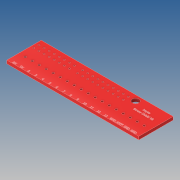
# Autodesk Inventor part: Arduino UNO R3 screw shield v2 board Left
Saved by Autodesk Inventor 2017 SP1 (Build 210196100, 196)
## iProperties
Created: 2022-11-07
Part Number: Arduino UNO R3 screw shield v2 board Left
Material: Generic
Document SubType Name: Modeling
Designer: Antonio
Density: 1 g/cm^3
Appearance: Rojo claro
Author: Antonio
Autodesk Inventor part; units mm, degrees
(part 1 of 2)
ref_plane "YZ Plane" through (0, 0, 0) normal (1, 0, 0) x (0, 1, 0)
ref_plane "XZ Plane" through (0, 0, 0) normal (0, 1, 0) x (-1, 0, 0)
ref_plane "XY Plane" through (0, 0, 0) normal (0, 0, 1) x (1, 0, 0)
sketch "Boceto1" plane through (0, 0, 0) normal (0, 0, 1) x (1, 0, 0)
  line L0 (0, 0) -> (66, 0)
  line L1 (66, 0) -> (66, 17.2)
  line L2 (66, 17.2) -> (0, 17.2)
  line L3 (0, 17.2) -> (0, 0)
  line L4 (0, 6) -> (66, 6) construction
  line L5 (3.3, 0) -> (3.3, 6) construction
  line L6 (6.8, 0) -> (6.8, 6) construction
  line L7 (10.3, 0) -> (10.3, 6) construction
  line L8 (13.8, 0) -> (13.8, 6) construction
  line L9 (17.3, 0) -> (17.3, 6) construction
  line L10 (20.8, 0) -> (20.8, 6) construction
  line L11 (24.3, 0) -> (24.3, 6) construction
  line L12 (27.8, 0) -> (27.8, 6) construction
  line L13 (31.3, 0) -> (31.3, 6) construction
  line L14 (34.8, 0) -> (34.8, 6) construction
  line L15 (38.3, 0) -> (38.3, 6) construction
  line L16 (41.8, 0) -> (41.8, 6) construction
  line L17 (45.3, 0) -> (45.3, 6) construction
  line L18 (48.8, 0) -> (48.8, 6) construction
  line L19 (52.3, 0) -> (52.3, 6) construction
  line L20 (55.8, 0) -> (55.8, 6) construction
  line L21 (59.3, 0) -> (59.3, 6) construction
  line L22 (62.8, 0) -> (62.8, 6) construction
  circle A0 centre (3.3, 6) radius 0.55
  circle A1 centre (6.8, 6) radius 0.55
  circle A2 centre (10.3, 6) radius 0.55
  circle A3 centre (13.8, 6) radius 0.55
  circle A4 centre (17.3, 6) radius 0.55
  circle A5 centre (20.8, 6) radius 0.55
  circle A6 centre (24.3, 6) radius 0.55
  circle A7 centre (27.8, 6) radius 0.55
  circle A8 centre (31.3, 6) radius 0.55
  circle A9 centre (34.8, 6) radius 0.55
  circle A10 centre (38.3, 6) radius 0.55
  circle A11 centre (41.8, 6) radius 0.55
  circle A12 centre (45.3, 6) radius 0.55
  circle A13 centre (48.8, 6) radius 0.55
  circle A14 centre (52.3, 6) radius 0.55
  circle A15 centre (55.8, 6) radius 0.55
  circle A16 centre (59.3, 6) radius 0.55
  circle A17 centre (62.8, 6) radius 0.55
  line L23 (0, 12) -> (66, 12) construction
  line L24 (0, 14.54) -> (66, 14.54) construction
  line L25 (1.54, 0) -> (1.54, 17.2) construction
  circle A18 centre (1.54, 14.54) radius 0.4
  circle A19 centre (4.08, 14.54) radius 0.4
  circle A20 centre (6.62, 14.54) radius 0.4
  circle A21 centre (9.16, 14.54) radius 0.4
  circle A22 centre (11.7, 14.54) radius 0.4
  circle A23 centre (14.24, 14.54) radius 0.4
  circle A24 centre (16.78, 14.54) radius 0.4
  circle A25 centre (19.32, 14.54) radius 0.4
  circle A26 centre (1.54, 12) radius 0.4
  circle A27 centre (4.08, 12) radius 0.4
  circle A28 centre (6.62, 12) radius 0.4
  circle A29 centre (9.16, 12) radius 0.4
  circle A30 centre (11.7, 12) radius 0.4
  circle A31 centre (14.24, 12) radius 0.4
  circle A32 centre (16.78, 12) radius 0.4
  circle A33 centre (19.32, 12) radius 0.4
  line L26 (19.32, 12) -> (19.32, 17.2) construction
  line L27 (23.384, 12) -> (23.384, 16.5) construction
  circle A34 centre (23.384, 14.54) radius 0.4
  circle A35 centre (25.924, 14.54) radius 0.4
  circle A36 centre (28.464, 14.54) radius 0.4
  circle A37 centre (31.004, 14.54) radius 0.4
  circle A38 centre (33.544, 14.54) radius 0.4
  circle A39 centre (36.084, 14.54) radius 0.4
  circle A40 centre (38.624, 14.54) radius 0.4
  circle A41 centre (41.164, 14.54) radius 0.4
  circle A42 centre (43.704, 14.54) radius 0.4
  circle A43 centre (46.244, 14.54) radius 0.4
  circle A44 centre (23.384, 12) radius 0.4
  circle A45 centre (25.924, 12) radius 0.4
  circle A46 centre (28.464, 12) radius 0.4
  circle A47 centre (31.004, 12) radius 0.4
  circle A48 centre (33.544, 12) radius 0.4
  circle A49 centre (36.084, 12) radius 0.4
  circle A50 centre (38.624, 12) radius 0.4
  circle A51 centre (41.164, 12) radius 0.4
  circle A52 centre (43.704, 12) radius 0.4
  circle A53 centre (46.244, 12) radius 0.4
  line L28 (46.244, 12) -> (46.244, 17.2) construction
  line L29 (50.76, 12) -> (50.76, 16.5) construction
  circle A54 centre (49.9, 14.54) radius 1.7
  line L30 (0, 0.2) -> (66, 0.2) construction
  line L31 (2.4235, 1.1897) -> (4.0751, 1.1897) construction
  line L32 (4.0751, 1.1897) -> (4.0751, 0.1897) construction
  line L33 (4.0751, 0.1897) -> (2.4235, 0.1897) construction
  line L34 (2.4235, 0.1897) -> (2.4235, 1.1897) construction
  line L35 (5.9424, 1.2002) -> (7.594, 1.2002) construction
  line L36 (7.594, 1.2002) -> (7.594, 0.2002) construction
  line L37 (7.594, 0.2002) -> (5.9424, 0.2002) construction
  line L38 (5.9424, 0.2002) -> (5.9424, 1.2002) construction
  line L39 (9.8961, 1.2406) -> (11.5477, 1.2406) construction
  line L40 (11.5477, 1.2406) -> (11.5477, 0.2406) construction
  line L41 (11.5477, 0.2406) -> (9.8961, 0.2406) construction
  line L42 (9.8961, 0.2406) -> (9.8961, 1.2406) construction
  line L43 (13.46, 0.221) -> (13.46, 1.221) construction
  line L44 (13.46, 1.221) -> (15.1116, 1.221) construction
  line L45 (15.1116, 1.221) -> (15.1116, 0.221) construction
  line L46 (15.1116, 0.221) -> (13.46, 0.221) construction
  line L47 (16.9339, 0.2315) -> (16.9339, 1.2315) construction
  line L48 (16.9339, 1.2315) -> (18.5855, 1.2315) construction
  line L49 (18.5855, 1.2315) -> (18.5855, 0.2315) construction
  line L50 (18.5855, 0.2315) -> (16.9339, 0.2315) construction
  line L51 (20.4229, 0.2269) -> (20.4229, 1.2269) construction
  line L52 (20.4229, 1.2269) -> (22.0744, 1.2269) construction
  line L53 (22.0744, 1.2269) -> (22.0744, 0.2269) construction
  line L54 (22.0744, 0.2269) -> (20.4229, 0.2269) construction
  line L55 (23.9268, 0.2373) -> (23.9268, 1.2373) construction
  line L56 (23.9268, 1.2373) -> (25.5783, 1.2373) construction
  line L57 (25.5783, 1.2373) -> (25.5783, 0.2373) construction
  line L58 (25.5783, 0.2373) -> (23.9268, 0.2373) construction
  line L59 (27.3857, 0.2627) -> (27.3857, 1.2627) construction
  line L60 (27.3857, 1.2627) -> (29.0372, 1.2627) construction
  line L61 (29.0372, 1.2627) -> (29.0372, 0.2627) construction
  line L62 (29.0372, 0.2627) -> (27.3857, 0.2627) construction
  line L63 (30.9196, 0.2732) -> (30.9196, 1.2732) construction
  line L64 (30.9196, 1.2732) -> (32.5711, 1.2732) construction
  line L65 (32.5711, 1.2732) -> (32.5711, 0.2732) construction
  line L66 (32.5711, 0.2732) -> (30.9196, 0.2732) construction
  line L67 (34.3935, 0.2386) -> (34.3935, 1.2386) construction
  line L68 (34.3935, 1.2386) -> (36.045, 1.2386) construction
  line L69 (36.045, 1.2386) -> (36.045, 0.2386) construction
  line L70 (36.045, 0.2386) -> (34.3935, 0.2386) construction
  line L71 (37.6275, 0.2041) -> (37.6275, 1.2041) construction
  line L72 (37.6275, 1.2041) -> (39.2791, 1.2041) construction
  line L73 (39.2791, 1.2041) -> (39.2791, 0.2041) construction
  line L74 (39.2791, 0.2041) -> (37.6275, 0.2041) construction
  line L75 (41.0265, 0.2295) -> (41.0265, 1.2295) construction
  line L76 (41.0265, 1.2295) -> (42.678, 1.2295) construction
  line L77 (42.678, 1.2295) -> (42.678, 0.2295) construction
  line L78 (42.678, 0.2295) -> (41.0265, 0.2295) construction
  line L79 (44.5754, 0.2249) -> (44.5754, 1.2249) construction
  line L80 (44.5754, 1.2249) -> (46.2269, 1.2249) construction
  line L81 (46.2269, 1.2249) -> (46.2269, 0.2249) construction
  line L82 (46.2269, 0.2249) -> (44.5754, 0.2249) construction
  line L83 (48.0793, 0.2204) -> (48.0793, 1.2204) construction
  line L84 (48.0793, 1.2204) -> (49.7308, 1.2204) construction
  line L85 (49.7308, 1.2204) -> (49.7308, 0.2204) construction
  line L86 (49.7308, 0.2204) -> (48.0793, 0.2204) construction
  line L87 (50.9534, 0.2458) -> (50.9534, 1.2458) construction
  line L88 (50.9534, 1.2458) -> (52.605, 1.2458) construction
  line L89 (52.605, 1.2458) -> (52.605, 0.2458) construction
  line L90 (52.605, 0.2458) -> (50.9534, 0.2458) construction
  line L91 (54.2025, 0.2263) -> (54.2025, 1.2263) construction
  line L92 (54.2025, 1.2263) -> (55.854, 1.2263) construction
  line L93 (55.854, 1.2263) -> (55.854, 0.2263) construction
  line L94 (55.854, 0.2263) -> (54.2025, 0.2263) construction
  line L95 (57.9208, 0.2413) -> (57.9208, 1.2413) construction
  line L96 (57.9208, 1.2413) -> (59.5724, 1.2413) construction
  line L97 (59.5724, 1.2413) -> (59.5724, 0.2413) construction
  line L98 (59.5724, 0.2413) -> (57.9208, 0.2413) construction
  line L99 (61.4098, 0.2067) -> (61.4098, 1.2067) construction
  line L100 (61.4098, 1.2067) -> (64.5007, 1.2067) construction
  line L101 (64.5007, 1.2067) -> (64.5007, 0.2067) construction
  line L102 (64.5007, 0.2067) -> (61.4098, 0.2067) construction
  line L103 (55.5956, 13.2313) -> (59.0259, 13.2313) construction
  line L104 (59.0259, 13.2313) -> (59.0259, 11.9104) construction
  line L105 (59.0259, 11.9104) -> (55.5956, 11.9104) construction
  line L106 (55.5956, 11.9104) -> (55.5956, 13.2313) construction
  line L107 (52.8192, 11.2798) -> (62.9552, 11.2798) construction
  line L108 (62.9552, 11.2798) -> (62.9552, 10.186) construction
  line L109 (62.9552, 10.186) -> (52.8192, 10.186) construction
  line L110 (52.8192, 10.186) -> (52.8192, 11.2798) construction
  line L111 (56.3087, 12.1867) -> (56.1426, 12.1867)
  line L112 (56.1426, 12.1867) -> (55.8638, 12.549)
  line L113 (55.8638, 12.549) -> (55.8136, 12.5004)
  line L114 (55.8136, 12.5004) -> (55.8136, 12.1867)
  line L115 (55.8136, 12.1867) -> (55.6872, 12.1867)
  line L116 (55.6872, 12.1867) -> (55.6872, 13.2313)
  line L117 (55.6872, 13.2313) -> (55.8136, 13.2313)
  line L118 (55.8136, 13.2313) -> (55.8136, 12.6203)
  line L119 (55.8136, 12.6203) -> (56.1102, 12.9371)
  line L120 (56.1102, 12.9371) -> (56.2674, 12.9371)
  line L121 (56.2674, 12.9371) -> (55.9595, 12.6235)
  line L122 (55.9595, 12.6235) -> (56.3087, 12.1867)
  spline S0 degree 2 poles (56.6977, 12.1697) (56.5178, 12.1697) (56.3201, 12.3715) (56.3201, 12.5579) knots 0 0 0 1 2 2 2
  spline S1 degree 2 poles (56.3201, 12.5579) (56.3201, 12.741) (56.5121, 12.9582) (56.6669, 12.9582) knots 0 0 0 1 2 2 2
  spline S2 degree 2 poles (56.6669, 12.9582) (56.7366, 12.9582) (56.8444, 12.9177) (56.8841, 12.8747) knots 0 0 0 1 2 2 2
  spline S3 degree 2 poles (56.8841, 12.8747) (56.9246, 12.8318) (56.9676, 12.7078) (56.9676, 12.6179) knots 0 0 0 1 2 2 2
  line L123 (56.9676, 12.6179) -> (56.9676, 12.549)
  line L124 (56.9676, 12.549) -> (56.4481, 12.549)
  spline S4 degree 2 poles (56.4481, 12.549) (56.4481, 12.4185) (56.5794, 12.2799) (56.6961, 12.2799) knots 0 0 0 1 2 2 2
  spline S5 degree 2 poles (56.6961, 12.2799) (56.7374, 12.2799) (56.8176, 12.2986) (56.8501, 12.3132) knots 0 0 0 1 2 2 2
  spline S6 degree 2 poles (56.8501, 12.3132) (56.8841, 12.3294) (56.9311, 12.3577) (56.9465, 12.3707) knots 0 0 0 1 2 2 2
  line L125 (56.9465, 12.3707) -> (56.9538, 12.3707)
  line L126 (56.9538, 12.3707) -> (56.9538, 12.2329)
  spline S7 degree 2 poles (56.9538, 12.2329) (56.9319, 12.224) (56.8655, 12.1981) (56.8395, 12.1908) knots 0 0 0 1 2 2 2
  spline S8 degree 2 poles (56.8395, 12.1908) (56.8031, 12.1803) (56.7431, 12.1697) (56.6977, 12.1697) knots 0 0 0 1 2 2 2
  spline S9 degree 2 poles (56.8444, 12.6454) (56.8428, 12.6965) (56.8217, 12.771) (56.8014, 12.7961) knots 0 0 0 1 2 2 2
  spline S10 degree 2 poles (56.8014, 12.7961) (56.7796, 12.8245) (56.7107, 12.8545) (56.6596, 12.8545) knots 0 0 0 1 2 2 2
  spline S11 degree 2 poles (56.6596, 12.8545) (56.6094, 12.8545) (56.5389, 12.8245) (56.5097, 12.7953) knots 0 0 0 1 2 2 2
  spline S12 degree 2 poles (56.5097, 12.7953) (56.4813, 12.7653) (56.4522, 12.6932) (56.4481, 12.6454) knots 0 0 0 1 2 2 2
  line L127 (56.4481, 12.6454) -> (56.8444, 12.6454)
  line L128 (57.6847, 12.9371) -> (57.2812, 11.9104)
  line L129 (57.2812, 11.9104) -> (57.1458, 11.9104)
  line L130 (57.1458, 11.9104) -> (57.2804, 12.2232)
  line L131 (57.2804, 12.2232) -> (57.0081, 12.9371)
  line L132 (57.0081, 12.9371) -> (57.1442, 12.9371)
  line L133 (57.1442, 12.9371) -> (57.3492, 12.3812)
  line L134 (57.3492, 12.3812) -> (57.5535, 12.9371)
  line L135 (57.5535, 12.9371) -> (57.6847, 12.9371)
  spline S13 degree 2 poles (58.1061, 12.1697) (57.9262, 12.1697) (57.7285, 12.3715) (57.7285, 12.5579) knots 0 0 0 1 2 2 2
  spline S14 degree 2 poles (57.7285, 12.5579) (57.7285, 12.741) (57.9206, 12.9582) (58.0753, 12.9582) knots 0 0 0 1 2 2 2
  spline S15 degree 2 poles (58.0753, 12.9582) (58.145, 12.9582) (58.2528, 12.9177) (58.2925, 12.8747) knots 0 0 0 1 2 2 2
  spline S16 degree 2 poles (58.2925, 12.8747) (58.333, 12.8318) (58.376, 12.7078) (58.376, 12.6179) knots 0 0 0 1 2 2 2
  line L136 (58.376, 12.6179) -> (58.376, 12.549)
  line L137 (58.376, 12.549) -> (57.8565, 12.549)
  spline S17 degree 2 poles (57.8565, 12.549) (57.8565, 12.4185) (57.9878, 12.2799) (58.1045, 12.2799) knots 0 0 0 1 2 2 2
  spline S18 degree 2 poles (58.1045, 12.2799) (58.1458, 12.2799) (58.2261, 12.2986) (58.2585, 12.3132) knots 0 0 0 1 2 2 2
  spline S19 degree 2 poles (58.2585, 12.3132) (58.2925, 12.3294) (58.3395, 12.3577) (58.3549, 12.3707) knots 0 0 0 1 2 2 2
  line L138 (58.3549, 12.3707) -> (58.3622, 12.3707)
  line L139 (58.3622, 12.3707) -> (58.3622, 12.2329)
  spline S20 degree 2 poles (58.3622, 12.2329) (58.3403, 12.224) (58.2739, 12.1981) (58.248, 12.1908) knots 0 0 0 1 2 2 2
  spline S21 degree 2 poles (58.248, 12.1908) (58.2115, 12.1803) (58.1515, 12.1697) (58.1061, 12.1697) knots 0 0 0 1 2 2 2
  spline S22 degree 2 poles (58.2528, 12.6454) (58.2512, 12.6965) (58.2301, 12.771) (58.2099, 12.7961) knots 0 0 0 1 2 2 2
  spline S23 degree 2 poles (58.2099, 12.7961) (58.188, 12.8245) (58.1191, 12.8545) (58.0681, 12.8545) knots 0 0 0 1 2 2 2
  spline S24 degree 2 poles (58.0681, 12.8545) (58.0178, 12.8545) (57.9473, 12.8245) (57.9181, 12.7953) knots 0 0 0 1 2 2 2
  spline S25 degree 2 poles (57.9181, 12.7953) (57.8898, 12.7653) (57.8606, 12.6932) (57.8565, 12.6454) knots 0 0 0 1 2 2 2
  line L140 (57.8565, 12.6454) -> (58.2528, 12.6454)
  spline S26 degree 2 poles (58.7066, 12.1689) (58.6313, 12.1689) (58.5008, 12.2094) (58.4578, 12.2321) knots 0 0 0 1 2 2 2
  line L141 (58.4578, 12.2321) -> (58.4578, 12.3739)
  line L142 (58.4578, 12.3739) -> (58.4643, 12.3739)
  spline S27 degree 2 poles (58.4643, 12.3739) (58.4805, 12.361) (58.5243, 12.3302) (58.5608, 12.3132) knots 0 0 0 1 2 2 2
  spline S28 degree 2 poles (58.5608, 12.3132) (58.5924, 12.2978) (58.6702, 12.2751) (58.7115, 12.2751) knots 0 0 0 1 2 2 2
  spline S29 degree 2 poles (58.7115, 12.2751) (58.7415, 12.2751) (58.8104, 12.2888) (58.8266, 12.3002) knots 0 0 0 1 2 2 2
  spline S30 degree 2 poles (58.8266, 12.3002) (58.8501, 12.3156) (58.8711, 12.3504) (58.8711, 12.3861) knots 0 0 0 1 2 2 2
  spline S31 degree 2 poles (58.8711, 12.3861) (58.8711, 12.4307) (58.8225, 12.4769) (58.7601, 12.4923) knots 0 0 0 1 2 2 2
  spline S32 degree 2 poles (58.7601, 12.4923) (58.7358, 12.4979) (58.658, 12.5141) (58.6248, 12.523) knots 0 0 0 1 2 2 2
  spline S33 degree 2 poles (58.6248, 12.523) (58.5389, 12.5482) (58.4611, 12.6519) (58.4611, 12.7256) knots 0 0 0 1 2 2 2
  spline S34 degree 2 poles (58.4611, 12.7256) (58.4611, 12.8277) (58.6142, 12.955) (58.7407, 12.955) knots 0 0 0 1 2 2 2
  spline S35 degree 2 poles (58.7407, 12.955) (58.8031, 12.955) (58.9295, 12.9242) (58.9724, 12.9007) knots 0 0 0 1 2 2 2
  line L143 (58.9724, 12.9007) -> (58.9724, 12.7653)
  line L144 (58.9724, 12.7653) -> (58.9659, 12.7653)
  spline S36 degree 2 poles (58.9659, 12.7653) (58.9173, 12.8042) (58.799, 12.8488) (58.7382, 12.8488) knots 0 0 0 1 2 2 2
  spline S37 degree 2 poles (58.7382, 12.8488) (58.6758, 12.8488) (58.5899, 12.7961) (58.5899, 12.7435) knots 0 0 0 1 2 2 2
  spline S38 degree 2 poles (58.5899, 12.7435) (58.5899, 12.6957) (58.641, 12.6495) (58.6977, 12.6349) knots 0 0 0 1 2 2 2
  spline S39 degree 2 poles (58.6977, 12.6349) (58.7253, 12.6276) (58.795, 12.613) (58.833, 12.6041) knots 0 0 0 1 2 2 2
  spline S40 degree 2 poles (58.833, 12.6041) (58.9157, 12.583) (59, 12.4866) (59, 12.4031) knots 0 0 0 1 2 2 2
  spline S41 degree 2 poles (59, 12.4031) (59, 12.3545) (58.9619, 12.2686) (58.9246, 12.237) knots 0 0 0 1 2 2 2
  spline S42 degree 2 poles (58.9246, 12.237) (58.8849, 12.2038) (58.7836, 12.1689) (58.7066, 12.1689) knots 0 0 0 1 2 2 2
  spline S43 degree 2 poles (53.1993, 10.2174) (53.0907, 10.2174) (52.9383, 10.2627) (52.8711, 10.2952) knots 0 0 0 1 2 2 2
  line L145 (52.8711, 10.2952) -> (52.8711, 10.4621)
  line L146 (52.8711, 10.4621) -> (52.8808, 10.4621)
  spline S44 degree 2 poles (52.8808, 10.4621) (52.9464, 10.4005) (53.1126, 10.3324) (53.1895, 10.3324) knots 0 0 0 1 2 2 2
  spline S45 degree 2 poles (53.1895, 10.3324) (53.2998, 10.3324) (53.4124, 10.424) (53.4124, 10.4994) knots 0 0 0 1 2 2 2
  spline S46 degree 2 poles (53.4124, 10.4994) (53.4124, 10.5593) (53.3532, 10.6339) (53.2892, 10.6525) knots 0 0 0 1 2 2 2
  spline S47 degree 2 poles (53.2892, 10.6525) (53.243, 10.6655) (53.166, 10.6833) (53.1085, 10.6979) knots 0 0 0 1 2 2 2
  spline S48 degree 2 poles (53.1085, 10.6979) (53.0566, 10.7117) (52.9748, 10.753) (52.9432, 10.7862) knots 0 0 0 1 2 2 2
  spline S49 degree 2 poles (52.9432, 10.7862) (52.9124, 10.8195) (52.8784, 10.9086) (52.8784, 10.967) knots 0 0 0 1 2 2 2
  spline S50 degree 2 poles (52.8784, 10.967) (52.8784, 11.0885) (53.068, 11.253) (53.2147, 11.253) knots 0 0 0 1 2 2 2
  spline S51 degree 2 poles (53.2147, 11.253) (53.2989, 11.253) (53.4481, 11.2198) (53.5121, 11.1882) knots 0 0 0 1 2 2 2
  line L147 (53.5121, 11.1882) -> (53.5121, 11.0294)
  line L148 (53.5121, 11.0294) -> (53.5024, 11.0294)
  spline S52 degree 2 poles (53.5024, 11.0294) (53.4545, 11.0731) (53.3054, 11.1379) (53.2236, 11.1379) knots 0 0 0 1 2 2 2
  spline S53 degree 2 poles (53.2236, 11.1379) (53.1312, 11.1379) (53.0169, 11.0512) (53.0169, 10.9807) knots 0 0 0 1 2 2 2
  spline S54 degree 2 poles (53.0169, 10.9807) (53.0169, 10.9175) (53.0842, 10.8422) (53.1474, 10.8251) knots 0 0 0 1 2 2 2
  spline S55 degree 2 poles (53.1474, 10.8251) (53.1895, 10.8138) (53.3119, 10.7846) (53.3524, 10.7725) knots 0 0 0 1 2 2 2
  spline S56 degree 2 poles (53.3524, 10.7725) (53.4554, 10.7409) (53.551, 10.6136) (53.551, 10.5204) knots 0 0 0 1 2 2 2
  spline S57 degree 2 poles (53.551, 10.5204) (53.551, 10.4613) (53.5032, 10.3478) (53.4602, 10.3081) knots 0 0 0 1 2 2 2
  spline S58 degree 2 poles (53.4602, 10.3081) (53.4124, 10.2644) (53.2908, 10.2174) (53.1993, 10.2174) knots 0 0 0 1 2 2 2
  spline S59 degree 2 poles (53.9748, 10.2182) (53.897, 10.2182) (53.7682, 10.266) (53.722, 10.3146) knots 0 0 0 1 2 2 2
  spline S60 degree 2 poles (53.722, 10.3146) (53.6758, 10.3624) (53.6247, 10.5099) (53.6247, 10.6088) knots 0 0 0 1 2 2 2
  spline S61 degree 2 poles (53.6247, 10.6088) (53.6247, 10.7076) (53.6774, 10.8519) (53.722, 10.9005) knots 0 0 0 1 2 2 2
  spline S62 degree 2 poles (53.722, 10.9005) (53.7665, 10.9499) (53.8986, 11.0026) (53.9748, 11.0026) knots 0 0 0 1 2 2 2
  spline S63 degree 2 poles (53.9748, 11.0026) (54.0364, 11.0026) (54.1515, 10.9678) (54.196, 10.9451) knots 0 0 0 1 2 2 2
  line L149 (54.196, 10.9451) -> (54.196, 10.8033)
  line L150 (54.196, 10.8033) -> (54.1887, 10.8033)
  spline S64 degree 2 poles (54.1887, 10.8033) (54.175, 10.8146) (54.1328, 10.8438) (54.1028, 10.8592) knots 0 0 0 1 2 2 2
  spline S65 degree 2 poles (54.1028, 10.8592) (54.0761, 10.8721) (54.0048, 10.8924) (53.9724, 10.8924) knots 0 0 0 1 2 2 2
  spline S66 degree 2 poles (53.9724, 10.8924) (53.8743, 10.8924) (53.7552, 10.7441) (53.7552, 10.6088) knots 0 0 0 1 2 2 2
  spline S67 degree 2 poles (53.7552, 10.6088) (53.7552, 10.4767) (53.8703, 10.3284) (53.9724, 10.3284) knots 0 0 0 1 2 2 2
  spline S68 degree 2 poles (53.9724, 10.3284) (54.034, 10.3284) (54.1458, 10.3794) (54.1887, 10.4191) knots 0 0 0 1 2 2 2
  line L151 (54.1887, 10.4191) -> (54.196, 10.4191)
  line L152 (54.196, 10.4191) -> (54.196, 10.2773)
  spline S69 degree 2 poles (54.196, 10.2773) (54.1774, 10.2684) (54.1207, 10.2433) (54.098, 10.2376) knots 0 0 0 1 2 2 2
  spline S70 degree 2 poles (54.098, 10.2376) (54.0656, 10.2279) (54.0145, 10.2182) (53.9748, 10.2182) knots 0 0 0 1 2 2 2
  line L153 (54.709, 10.8503) -> (54.7025, 10.8503)
  spline S71 degree 2 poles (54.7025, 10.8503) (54.6879, 10.8543) (54.6563, 10.8559) (54.6344, 10.8559) knots 0 0 0 1 2 2 2
  spline S72 degree 2 poles (54.6344, 10.8559) (54.5834, 10.8559) (54.4829, 10.8114) (54.4375, 10.7676) knots 0 0 0 1 2 2 2
  line L154 (54.4375, 10.7676) -> (54.4375, 10.2352)
  line L155 (54.4375, 10.2352) -> (54.3111, 10.2352)
  line L156 (54.3111, 10.2352) -> (54.3111, 10.9856)
  line L157 (54.3111, 10.9856) -> (54.4375, 10.9856)
  line L158 (54.4375, 10.9856) -> (54.4375, 10.8738)
  spline S73 degree 2 poles (54.4375, 10.8738) (54.5064, 10.9353) (54.6093, 10.9856) (54.6579, 10.9856) knots 0 0 0 1 2 2 2
  spline S74 degree 2 poles (54.6579, 10.9856) (54.6774, 10.9856) (54.6968, 10.984) (54.709, 10.9815) knots 0 0 0 1 2 2 2
  line L159 (54.709, 10.9815) -> (54.709, 10.8503)
  spline S75 degree 2 poles (55.1328, 10.2182) (54.9529, 10.2182) (54.7552, 10.42) (54.7552, 10.6063) knots 0 0 0 1 2 2 2
  spline S76 degree 2 poles (54.7552, 10.6063) (54.7552, 10.7895) (54.9472, 11.0067) (55.102, 11.0067) knots 0 0 0 1 2 2 2
  spline S77 degree 2 poles (55.102, 11.0067) (55.1717, 11.0067) (55.2795, 10.9661) (55.3192, 10.9232) knots 0 0 0 1 2 2 2
  spline S78 degree 2 poles (55.3192, 10.9232) (55.3597, 10.8802) (55.4027, 10.7563) (55.4027, 10.6663) knots 0 0 0 1 2 2 2
  line L160 (55.4027, 10.6663) -> (55.4027, 10.5974)
  line L161 (55.4027, 10.5974) -> (54.8832, 10.5974)
  spline S79 degree 2 poles (54.8832, 10.5974) (54.8832, 10.467) (55.0145, 10.3284) (55.1312, 10.3284) knots 0 0 0 1 2 2 2
  spline S80 degree 2 poles (55.1312, 10.3284) (55.1725, 10.3284) (55.2528, 10.347) (55.2852, 10.3616) knots 0 0 0 1 2 2 2
  spline S81 degree 2 poles (55.2852, 10.3616) (55.3192, 10.3778) (55.3662, 10.4062) (55.3816, 10.4191) knots 0 0 0 1 2 2 2
  line L162 (55.3816, 10.4191) -> (55.3889, 10.4191)
  line L163 (55.3889, 10.4191) -> (55.3889, 10.2814)
  spline S82 degree 2 poles (55.3889, 10.2814) (55.367, 10.2725) (55.3006, 10.2465) (55.2746, 10.2392) knots 0 0 0 1 2 2 2
  spline S83 degree 2 poles (55.2746, 10.2392) (55.2382, 10.2287) (55.1782, 10.2182) (55.1328, 10.2182) knots 0 0 0 1 2 2 2
  spline S84 degree 2 poles (55.2795, 10.6939) (55.2779, 10.7449) (55.2568, 10.8195) (55.2366, 10.8446) knots 0 0 0 1 2 2 2
  spline S85 degree 2 poles (55.2366, 10.8446) (55.2147, 10.8729) (55.1458, 10.9029) (55.0947, 10.9029) knots 0 0 0 1 2 2 2
  spline S86 degree 2 poles (55.0947, 10.9029) (55.0445, 10.9029) (54.974, 10.8729) (54.9448, 10.8438) knots 0 0 0 1 2 2 2
  spline S87 degree 2 poles (54.9448, 10.8438) (54.9165, 10.8138) (54.8873, 10.7417) (54.8832, 10.6939) knots 0 0 0 1 2 2 2
  line L164 (54.8832, 10.6939) -> (55.2795, 10.6939)
  line L165 (56.44, 10.9856) -> (56.2495, 10.2352)
  line L166 (56.2495, 10.2352) -> (56.1328, 10.2352)
  line L167 (56.1328, 10.2352) -> (55.9497, 10.8138)
  line L168 (55.9497, 10.8138) -> (55.7673, 10.2352)
  line L169 (55.7673, 10.2352) -> (55.6515, 10.2352)
  line L170 (55.6515, 10.2352) -> (55.4594, 10.9856)
  line L171 (55.4594, 10.9856) -> (55.5907, 10.9856)
  line L172 (55.5907, 10.9856) -> (55.7236, 10.4046)
  line L173 (55.7236, 10.4046) -> (55.9011, 10.9856)
  line L174 (55.9011, 10.9856) -> (56.0056, 10.9856)
  line L175 (56.0056, 10.9856) -> (56.1879, 10.4046)
  line L176 (56.1879, 10.4046) -> (56.3127, 10.9856)
  line L177 (56.3127, 10.9856) -> (56.44, 10.9856)
  spline S88 degree 2 poles (57.269, 10.2174) (57.1604, 10.2174) (57.008, 10.2627) (56.9408, 10.2952) knots 0 0 0 1 2 2 2
  line L178 (56.9408, 10.2952) -> (56.9408, 10.4621)
  line L179 (56.9408, 10.4621) -> (56.9505, 10.4621)
  spline S89 degree 2 poles (56.9505, 10.4621) (57.0161, 10.4005) (57.1823, 10.3324) (57.2592, 10.3324) knots 0 0 0 1 2 2 2
  spline S90 degree 2 poles (57.2592, 10.3324) (57.3695, 10.3324) (57.4821, 10.424) (57.4821, 10.4994) knots 0 0 0 1 2 2 2
  spline S91 degree 2 poles (57.4821, 10.4994) (57.4821, 10.5593) (57.4229, 10.6339) (57.3589, 10.6525) knots 0 0 0 1 2 2 2
  spline S92 degree 2 poles (57.3589, 10.6525) (57.3127, 10.6655) (57.2357, 10.6833) (57.1782, 10.6979) knots 0 0 0 1 2 2 2
  spline S93 degree 2 poles (57.1782, 10.6979) (57.1263, 10.7117) (57.0445, 10.753) (57.0129, 10.7862) knots 0 0 0 1 2 2 2
  spline S94 degree 2 poles (57.0129, 10.7862) (56.9821, 10.8195) (56.9481, 10.9086) (56.9481, 10.967) knots 0 0 0 1 2 2 2
  spline S95 degree 2 poles (56.9481, 10.967) (56.9481, 11.0885) (57.1377, 11.253) (57.2844, 11.253) knots 0 0 0 1 2 2 2
  spline S96 degree 2 poles (57.2844, 11.253) (57.3686, 11.253) (57.5177, 11.2198) (57.5818, 11.1882) knots 0 0 0 1 2 2 2
  line L180 (57.5818, 11.1882) -> (57.5818, 11.0294)
  line L181 (57.5818, 11.0294) -> (57.572, 11.0294)
  spline S97 degree 2 poles (57.572, 11.0294) (57.5242, 11.0731) (57.3751, 11.1379) (57.2933, 11.1379) knots 0 0 0 1 2 2 2
  spline S98 degree 2 poles (57.2933, 11.1379) (57.2009, 11.1379) (57.0866, 11.0512) (57.0866, 10.9807) knots 0 0 0 1 2 2 2
  spline S99 degree 2 poles (57.0866, 10.9807) (57.0866, 10.9175) (57.1539, 10.8422) (57.2171, 10.8251) knots 0 0 0 1 2 2 2
  spline S100 degree 2 poles (57.2171, 10.8251) (57.2592, 10.8138) (57.3816, 10.7846) (57.4221, 10.7725) knots 0 0 0 1 2 2 2
  spline S101 degree 2 poles (57.4221, 10.7725) (57.525, 10.7409) (57.6207, 10.6136) (57.6207, 10.5204) knots 0 0 0 1 2 2 2
  spline S102 degree 2 poles (57.6207, 10.5204) (57.6207, 10.4613) (57.5729, 10.3478) (57.5299, 10.3081) knots 0 0 0 1 2 2 2
  spline S103 degree 2 poles (57.5299, 10.3081) (57.4821, 10.2644) (57.3605, 10.2174) (57.269, 10.2174) knots 0 0 0 1 2 2 2
  line L182 (58.3354, 10.2352) -> (58.209, 10.2352)
  line L183 (58.209, 10.2352) -> (58.209, 10.6631)
  spline S104 degree 2 poles (58.209, 10.6631) (58.209, 10.7149) (58.1993, 10.8041) (58.1847, 10.8308) knots 0 0 0 1 2 2 2
  spline S105 degree 2 poles (58.1847, 10.8308) (58.1693, 10.8592) (58.1142, 10.8867) (58.0672, 10.8867) knots 0 0 0 1 2 2 2
  spline S106 degree 2 poles (58.0672, 10.8867) (58.0202, 10.8867) (57.9205, 10.8365) (57.8727, 10.796) knots 0 0 0 1 2 2 2
  line L184 (57.8727, 10.796) -> (57.8727, 10.2352)
  line L185 (57.8727, 10.2352) -> (57.7463, 10.2352)
  line L186 (57.7463, 10.2352) -> (57.7463, 11.2798)
  line L187 (57.7463, 11.2798) -> (57.8727, 11.2798)
  line L188 (57.8727, 11.2798) -> (57.8727, 10.9021)
  spline S107 degree 2 poles (57.8727, 10.9021) (57.9294, 10.9532) (58.0388, 11.0067) (58.1004, 11.0067) knots 0 0 0 1 2 2 2
  spline S108 degree 2 poles (58.1004, 11.0067) (58.2106, 11.0067) (58.3354, 10.8608) (58.3354, 10.7222) knots 0 0 0 1 2 2 2
  line L189 (58.3354, 10.7222) -> (58.3354, 10.2352)
  line L190 (58.6417, 10.2352) -> (58.5153, 10.2352)
  line L191 (58.5153, 10.2352) -> (58.5153, 10.9856)
  line L192 (58.5153, 10.9856) -> (58.6417, 10.9856)
  line L193 (58.6417, 10.9856) -> (58.6417, 10.2352)
  line L194 (58.6507, 11.1104) -> (58.5072, 11.1104)
  line L195 (58.5072, 11.1104) -> (58.5072, 11.2417)
  line L196 (58.5072, 11.2417) -> (58.6507, 11.2417)
  line L197 (58.6507, 11.2417) -> (58.6507, 11.1104)
  spline S109 degree 2 poles (59.1531, 10.2182) (58.9732, 10.2182) (58.7754, 10.42) (58.7754, 10.6063) knots 0 0 0 1 2 2 2
  spline S110 degree 2 poles (58.7754, 10.6063) (58.7754, 10.7895) (58.9675, 11.0067) (59.1223, 11.0067) knots 0 0 0 1 2 2 2
  spline S111 degree 2 poles (59.1223, 11.0067) (59.192, 11.0067) (59.2998, 10.9661) (59.3395, 10.9232) knots 0 0 0 1 2 2 2
  spline S112 degree 2 poles (59.3395, 10.9232) (59.38, 10.8802) (59.4229, 10.7563) (59.4229, 10.6663) knots 0 0 0 1 2 2 2
  line L198 (59.4229, 10.6663) -> (59.4229, 10.5974)
  line L199 (59.4229, 10.5974) -> (58.9035, 10.5974)
  spline S113 degree 2 poles (58.9035, 10.5974) (58.9035, 10.467) (59.0348, 10.3284) (59.1515, 10.3284) knots 0 0 0 1 2 2 2
  spline S114 degree 2 poles (59.1515, 10.3284) (59.1928, 10.3284) (59.273, 10.347) (59.3054, 10.3616) knots 0 0 0 1 2 2 2
  spline S115 degree 2 poles (59.3054, 10.3616) (59.3395, 10.3778) (59.3865, 10.4062) (59.4019, 10.4191) knots 0 0 0 1 2 2 2
  line L200 (59.4019, 10.4191) -> (59.4092, 10.4191)
  line L201 (59.4092, 10.4191) -> (59.4092, 10.2814)
  spline S116 degree 2 poles (59.4092, 10.2814) (59.3873, 10.2725) (59.3208, 10.2465) (59.2949, 10.2392) knots 0 0 0 1 2 2 2
  spline S117 degree 2 poles (59.2949, 10.2392) (59.2584, 10.2287) (59.1985, 10.2182) (59.1531, 10.2182) knots 0 0 0 1 2 2 2
  spline S118 degree 2 poles (59.2998, 10.6939) (59.2981, 10.7449) (59.2771, 10.8195) (59.2568, 10.8446) knots 0 0 0 1 2 2 2
  spline S119 degree 2 poles (59.2568, 10.8446) (59.2349, 10.8729) (59.166, 10.9029) (59.115, 10.9029) knots 0 0 0 1 2 2 2
  spline S120 degree 2 poles (59.115, 10.9029) (59.0648, 10.9029) (58.9942, 10.8729) (58.9651, 10.8438) knots 0 0 0 1 2 2 2
  spline S121 degree 2 poles (58.9651, 10.8438) (58.9367, 10.8138) (58.9075, 10.7417) (58.9035, 10.6939) knots 0 0 0 1 2 2 2
  line L202 (58.9035, 10.6939) -> (59.2998, 10.6939)
  line L203 (59.6798, 10.2352) -> (59.5534, 10.2352)
  line L204 (59.5534, 10.2352) -> (59.5534, 11.2798)
  line L205 (59.5534, 11.2798) -> (59.6798, 11.2798)
  line L206 (59.6798, 11.2798) -> (59.6798, 10.2352)
  line L207 (60.4424, 10.2352) -> (60.316, 10.2352)
  line L208 (60.316, 10.2352) -> (60.316, 10.3114)
  spline S122 degree 2 poles (60.316, 10.3114) (60.2868, 10.2871) (60.2438, 10.2546) (60.2147, 10.2409) knots 0 0 0 1 2 2 2
  spline S123 degree 2 poles (60.2147, 10.2409) (60.1879, 10.2279) (60.1304, 10.2141) (60.0923, 10.2141) knots 0 0 0 1 2 2 2
  spline S124 degree 2 poles (60.0923, 10.2141) (60.0307, 10.2141) (59.927, 10.2652) (59.8905, 10.3146) knots 0 0 0 1 2 2 2
  spline S125 degree 2 poles (59.8905, 10.3146) (59.8541, 10.364) (59.8135, 10.5099) (59.8135, 10.6047) knots 0 0 0 1 2 2 2
  spline S126 degree 2 poles (59.8135, 10.6047) (59.8135, 10.7036) (59.8646, 10.8478) (59.9092, 10.9021) knots 0 0 0 1 2 2 2
  spline S127 degree 2 poles (59.9092, 10.9021) (59.9505, 10.9507) (60.0664, 11.0067) (60.1304, 11.0067) knots 0 0 0 1 2 2 2
  spline S128 degree 2 poles (60.1304, 11.0067) (60.1863, 11.0067) (60.2698, 10.9815) (60.316, 10.9556) knots 0 0 0 1 2 2 2
  line L209 (60.316, 10.9556) -> (60.316, 11.2798)
  line L210 (60.316, 11.2798) -> (60.4424, 11.2798)
  line L211 (60.4424, 11.2798) -> (60.4424, 10.2352)
  line L212 (60.316, 10.4175) -> (60.316, 10.8511)
  spline S129 degree 2 poles (60.316, 10.8511) (60.269, 10.8738) (60.1944, 10.8908) (60.1515, 10.8908) knots 0 0 0 1 2 2 2
  spline S130 degree 2 poles (60.1515, 10.8908) (60.0542, 10.8908) (59.944, 10.7449) (59.944, 10.6071) knots 0 0 0 1 2 2 2
  spline S131 degree 2 poles (59.944, 10.6071) (59.944, 10.4742) (60.0283, 10.3341) (60.1215, 10.3341) knots 0 0 0 1 2 2 2
  spline S132 degree 2 poles (60.1215, 10.3341) (60.1709, 10.3341) (60.2714, 10.3794) (60.316, 10.4175) knots 0 0 0 1 2 2 2
  line L213 (61.79, 11.2352) -> (61.4456, 10.2352)
  line L214 (61.4456, 10.2352) -> (61.3022, 10.2352)
  line L215 (61.3022, 10.2352) -> (60.9578, 11.2352)
  line L216 (60.9578, 11.2352) -> (61.1004, 11.2352)
  line L217 (61.1004, 11.2352) -> (61.3776, 10.4046)
  line L218 (61.3776, 10.4046) -> (61.6547, 11.2352)
  line L219 (61.6547, 11.2352) -> (61.79, 11.2352)
  line L220 (62.474, 10.2352) -> (61.8573, 10.2352)
  line L221 (61.8573, 10.2352) -> (61.8573, 10.377)
  spline S133 degree 2 poles (61.8573, 10.377) (61.9237, 10.4394) (62.0421, 10.5553) (62.0988, 10.6177) knots 0 0 0 1 2 2 2
  spline S134 degree 2 poles (62.0988, 10.6177) (62.213, 10.7433) (62.2965, 10.894) (62.2965, 10.9742) knots 0 0 0 1 2 2 2
  spline S135 degree 2 poles (62.2965, 10.9742) (62.2965, 11.0164) (62.2706, 11.0796) (62.2471, 11.0999) knots 0 0 0 1 2 2 2
  spline S136 degree 2 poles (62.2471, 11.0999) (62.2236, 11.1201) (62.162, 11.1404) (62.1247, 11.1404) knots 0 0 0 1 2 2 2
  spline S137 degree 2 poles (62.1247, 11.1404) (62.0891, 11.1404) (62.0161, 11.1225) (61.9829, 11.1088) knots 0 0 0 1 2 2 2
  spline S138 degree 2 poles (61.9829, 11.1088) (61.9545, 11.0974) (61.9019, 11.065) (61.8857, 11.0537) knots 0 0 0 1 2 2 2
  line L222 (61.8857, 11.0537) -> (61.8784, 11.0537)
  line L223 (61.8784, 11.0537) -> (61.8784, 11.1963)
  spline S139 degree 2 poles (61.8784, 11.1963) (61.9197, 11.2165) (62.068, 11.2563) (62.1344, 11.2563) knots 0 0 0 1 2 2 2
  spline S140 degree 2 poles (62.1344, 11.2563) (62.2746, 11.2563) (62.4327, 11.108) (62.4327, 10.9815) knots 0 0 0 1 2 2 2
  spline S141 degree 2 poles (62.4327, 10.9815) (62.4327, 10.9224) (62.4051, 10.8235) (62.3808, 10.7814) knots 0 0 0 1 2 2 2
  spline S142 degree 2 poles (62.3808, 10.7814) (62.3565, 10.7376) (62.286, 10.6517) (62.2471, 10.6104) knots 0 0 0 1 2 2 2
  spline S143 degree 2 poles (62.2471, 10.6104) (62.1839, 10.5415) (62.0291, 10.394) (61.9829, 10.3511) knots 0 0 0 1 2 2 2
  line L224 (61.9829, 10.3511) -> (62.474, 10.3511)
  line L225 (62.474, 10.3511) -> (62.474, 10.2352)
  spline S144 degree 2 poles (61.93, 0.1694) (61.8239, 0.1694) (61.648, 0.2343) (61.5848, 0.2999) knots 0 0 0 1 2 2 2
  spline S145 degree 2 poles (61.5848, 0.2999) (61.5216, 0.3663) (61.4543, 0.5625) (61.4543, 0.6897) knots 0 0 0 1 2 2 2
  spline S146 degree 2 poles (61.4543, 0.6897) (61.4543, 0.8104) (61.5224, 1.0017) (61.5856, 1.0698) knots 0 0 0 1 2 2 2
  spline S147 degree 2 poles (61.5856, 1.0698) (61.6464, 1.1354) (61.8247, 1.2067) (61.9308, 1.2067) knots 0 0 0 1 2 2 2
  spline S148 degree 2 poles (61.9308, 1.2067) (61.9819, 1.2067) (62.0743, 1.1921) (62.1164, 1.1792) knots 0 0 0 1 2 2 2
  spline S149 degree 2 poles (62.1164, 1.1792) (62.1504, 1.1694) (62.2331, 1.1338) (62.2582, 1.1208) knots 0 0 0 1 2 2 2
  line L226 (62.2582, 1.1208) -> (62.2582, 0.9604)
  line L227 (62.2582, 0.9604) -> (62.2469, 0.9604)
  spline S150 degree 2 poles (62.2469, 0.9604) (62.2217, 0.9822) (62.1691, 1.0219) (62.1204, 1.0446) knots 0 0 0 1 2 2 2
  spline S151 degree 2 poles (62.1204, 1.0446) (62.0799, 1.0649) (61.9754, 1.0916) (61.9154, 1.0916) knots 0 0 0 1 2 2 2
  spline S152 degree 2 poles (61.9154, 1.0916) (61.7712, 1.0916) (61.5929, 0.8745) (61.5929, 0.6937) knots 0 0 0 1 2 2 2
  spline S153 degree 2 poles (61.5929, 0.6937) (61.5929, 0.5933) (61.6399, 0.4425) (61.6845, 0.3907) knots 0 0 0 1 2 2 2
  spline S154 degree 2 poles (61.6845, 0.3907) (61.7274, 0.3388) (61.849, 0.2845) (61.9251, 0.2845) knots 0 0 0 1 2 2 2
  spline S155 degree 2 poles (61.9251, 0.2845) (61.9811, 0.2845) (62.0929, 0.3007) (62.131, 0.3169) knots 0 0 0 1 2 2 2
  line L228 (62.131, 0.3169) -> (62.131, 0.5754)
  line L229 (62.131, 0.5754) -> (61.8992, 0.5754)
  line L230 (61.8992, 0.5754) -> (61.8992, 0.6921)
  line L231 (61.8992, 0.6921) -> (62.2623, 0.6921)
  line L232 (62.2623, 0.6921) -> (62.2623, 0.2553)
  spline S156 degree 2 poles (62.2623, 0.2553) (62.2371, 0.244) (62.1512, 0.2091) (62.1148, 0.1986) knots 0 0 0 1 2 2 2
  spline S157 degree 2 poles (62.1148, 0.1986) (62.0653, 0.184) (61.9859, 0.1694) (61.93, 0.1694) knots 0 0 0 1 2 2 2
  line L233 (63.1448, 0.1889) -> (62.9957, 0.1889)
  line L234 (62.9957, 0.1889) -> (62.5532, 1.0511)
  line L235 (62.5532, 1.0511) -> (62.5532, 0.1889)
  line L236 (62.5532, 0.1889) -> (62.4292, 0.1889)
  line L237 (62.4292, 0.1889) -> (62.4292, 1.1889)
  line L238 (62.4292, 1.1889) -> (62.618, 1.1889)
  line L239 (62.618, 1.1889) -> (63.0208, 0.3971)
  line L240 (63.0208, 0.3971) -> (63.0208, 1.1889)
  line L241 (63.0208, 1.1889) -> (63.1448, 1.1889)
  line L242 (63.1448, 1.1889) -> (63.1448, 0.1889)
  spline S158 degree 2 poles (64.1358, 0.6881) (64.1358, 0.5511) (64.0248, 0.3307) (63.9316, 0.2691) knots 0 0 0 1 2 2 2
  spline S159 degree 2 poles (63.9316, 0.2691) (63.8555, 0.2213) (63.6991, 0.1889) (63.5775, 0.1889) knots 0 0 0 1 2 2 2
  line L243 (63.5775, 0.1889) -> (63.3474, 0.1889)
  line L244 (63.3474, 0.1889) -> (63.3474, 1.1889)
  line L245 (63.3474, 1.1889) -> (63.5751, 1.1889)
  spline S160 degree 2 poles (63.5751, 1.1889) (63.7161, 1.1889) (63.8765, 1.1467) (63.9333, 1.1095) knots 0 0 0 1 2 2 2
  spline S161 degree 2 poles (63.9333, 1.1095) (64.0297, 1.0454) (64.1358, 0.8339) (64.1358, 0.6881) knots 0 0 0 1 2 2 2
  spline S162 degree 2 poles (63.9973, 0.6897) (63.9973, 0.8048) (63.9211, 0.9676) (63.8457, 1.0138) knots 0 0 0 1 2 2 2
  spline S163 degree 2 poles (63.8457, 1.0138) (63.7922, 1.0454) (63.6715, 1.0738) (63.5816, 1.0738) knots 0 0 0 1 2 2 2
  line L246 (63.5816, 1.0738) -> (63.4803, 1.0738)
  line L247 (63.4803, 1.0738) -> (63.4803, 0.304)
  line L248 (63.4803, 0.304) -> (63.5816, 0.304)
  spline S164 degree 2 poles (63.5816, 0.304) (63.6699, 0.304) (63.8036, 0.3323) (63.8579, 0.3704) knots 0 0 0 1 2 2 2
  spline S165 degree 2 poles (63.8579, 0.3704) (63.9276, 0.4174) (63.9973, 0.573) (63.9973, 0.6897) knots 0 0 0 1 2 2 2
  spline S166 degree 2 poles (58.4411, 0.204) (58.3349, 0.204) (58.1591, 0.2688) (58.0959, 0.3344) knots 0 0 0 1 2 2 2
  spline S167 degree 2 poles (58.0959, 0.3344) (58.0327, 0.4009) (57.9654, 0.597) (57.9654, 0.7242) knots 0 0 0 1 2 2 2
  spline S168 degree 2 poles (57.9654, 0.7242) (57.9654, 0.845) (58.0335, 1.0362) (58.0967, 1.1043) knots 0 0 0 1 2 2 2
  spline S169 degree 2 poles (58.0967, 1.1043) (58.1575, 1.1699) (58.3358, 1.2413) (58.4419, 1.2413) knots 0 0 0 1 2 2 2
  spline S170 degree 2 poles (58.4419, 1.2413) (58.493, 1.2413) (58.5853, 1.2267) (58.6275, 1.2137) knots 0 0 0 1 2 2 2
  spline S171 degree 2 poles (58.6275, 1.2137) (58.6615, 1.204) (58.7442, 1.1683) (58.7693, 1.1554) knots 0 0 0 1 2 2 2
  line L249 (58.7693, 1.1554) -> (58.7693, 0.9949)
  line L250 (58.7693, 0.9949) -> (58.758, 0.9949)
  spline S172 degree 2 poles (58.758, 0.9949) (58.7328, 1.0168) (58.6802, 1.0565) (58.6315, 1.0792) knots 0 0 0 1 2 2 2
  spline S173 degree 2 poles (58.6315, 1.0792) (58.591, 1.0994) (58.4865, 1.1262) (58.4265, 1.1262) knots 0 0 0 1 2 2 2
  spline S174 degree 2 poles (58.4265, 1.1262) (58.2823, 1.1262) (58.104, 0.909) (58.104, 0.7283) knots 0 0 0 1 2 2 2
  spline S175 degree 2 poles (58.104, 0.7283) (58.104, 0.6278) (58.151, 0.4771) (58.1956, 0.4252) knots 0 0 0 1 2 2 2
  spline S176 degree 2 poles (58.1956, 0.4252) (58.2385, 0.3733) (58.3601, 0.319) (58.4362, 0.319) knots 0 0 0 1 2 2 2
  spline S177 degree 2 poles (58.4362, 0.319) (58.4922, 0.319) (58.604, 0.3353) (58.6421, 0.3515) knots 0 0 0 1 2 2 2
  line L251 (58.6421, 0.3515) -> (58.6421, 0.61)
  line L252 (58.6421, 0.61) -> (58.4103, 0.61)
  line L253 (58.4103, 0.61) -> (58.4103, 0.7267)
  line L254 (58.4103, 0.7267) -> (58.7734, 0.7267)
  line L255 (58.7734, 0.7267) -> (58.7734, 0.2899)
  spline S178 degree 2 poles (58.7734, 0.2899) (58.7482, 0.2785) (58.6623, 0.2437) (58.6259, 0.2332) knots 0 0 0 1 2 2 2
  spline S179 degree 2 poles (58.6259, 0.2332) (58.5764, 0.2186) (58.497, 0.204) (58.4411, 0.204) knots 0 0 0 1 2 2 2
  line L256 (59.6558, 0.2234) -> (59.5067, 0.2234)
  line L257 (59.5067, 0.2234) -> (59.0643, 1.0857)
  line L258 (59.0643, 1.0857) -> (59.0643, 0.2234)
  line L259 (59.0643, 0.2234) -> (58.9403, 0.2234)
  line L260 (58.9403, 0.2234) -> (58.9403, 1.2234)
  line L261 (58.9403, 1.2234) -> (59.1291, 1.2234)
  line L262 (59.1291, 1.2234) -> (59.5319, 0.4317)
  line L263 (59.5319, 0.4317) -> (59.5319, 1.2234)
  line L264 (59.5319, 1.2234) -> (59.6558, 1.2234)
  line L265 (59.6558, 1.2234) -> (59.6558, 0.2234)
  spline S180 degree 2 poles (60.6469, 0.7226) (60.6469, 0.5857) (60.5359, 0.3652) (60.4427, 0.3037) knots 0 0 0 1 2 2 2
  spline S181 degree 2 poles (60.4427, 0.3037) (60.3665, 0.2558) (60.2101, 0.2234) (60.0886, 0.2234) knots 0 0 0 1 2 2 2
  line L266 (60.0886, 0.2234) -> (59.8584, 0.2234)
  line L267 (59.8584, 0.2234) -> (59.8584, 1.2234)
  line L268 (59.8584, 1.2234) -> (60.0862, 1.2234)
  spline S182 degree 2 poles (60.0862, 1.2234) (60.2272, 1.2234) (60.3876, 1.1813) (60.4443, 1.144) knots 0 0 0 1 2 2 2
  spline S183 degree 2 poles (60.4443, 1.144) (60.5408, 1.08) (60.6469, 0.8685) (60.6469, 0.7226) knots 0 0 0 1 2 2 2
  spline S184 degree 2 poles (60.5084, 0.7242) (60.5084, 0.8393) (60.4322, 1.0022) (60.3568, 1.0484) knots 0 0 0 1 2 2 2
  spline S185 degree 2 poles (60.3568, 1.0484) (60.3033, 1.08) (60.1826, 1.1084) (60.0926, 1.1084) knots 0 0 0 1 2 2 2
  line L269 (60.0926, 1.1084) -> (59.9913, 1.1084)
  line L270 (59.9913, 1.1084) -> (59.9913, 0.3385)
  line L271 (59.9913, 0.3385) -> (60.0926, 0.3385)
  spline S186 degree 2 poles (60.0926, 0.3385) (60.181, 0.3385) (60.3147, 0.3669) (60.369, 0.4049) knots 0 0 0 1 2 2 2
  spline S187 degree 2 poles (60.369, 0.4049) (60.4387, 0.452) (60.5084, 0.6075) (60.5084, 0.7242) knots 0 0 0 1 2 2 2
  line L272 (54.196, 0.2263) -> (54.5331, 1.2263)
  line L273 (54.5331, 1.2263) -> (54.6968, 1.2263)
  line L274 (54.6968, 1.2263) -> (55.0339, 0.2263)
  line L275 (55.0339, 0.2263) -> (54.8937, 0.2263)
  line L276 (54.8937, 0.2263) -> (54.803, 0.5058)
  line L277 (54.803, 0.5058) -> (54.4213, 0.5058)
  line L278 (54.4213, 0.5058) -> (54.3305, 0.2263)
  line L279 (54.3305, 0.2263) -> (54.196, 0.2263)
  line L280 (54.7665, 0.6193) -> (54.6117, 1.0901)
  line L281 (54.6117, 1.0901) -> (54.4577, 0.6193)
  line L282 (54.4577, 0.6193) -> (54.7665, 0.6193)
  line L283 (55.9026, 0.2263) -> (55.73, 0.2263)
  line L284 (55.73, 0.2263) -> (55.414, 0.6242)
  line L285 (55.414, 0.6242) -> (55.2616, 0.6242)
  line L286 (55.2616, 0.6242) -> (55.2616, 0.2263)
  line L287 (55.2616, 0.2263) -> (55.1287, 0.2263)
  line L288 (55.1287, 0.2263) -> (55.1287, 1.2263)
  line L289 (55.1287, 1.2263) -> (55.3864, 1.2263)
  spline S188 degree 2 poles (55.3864, 1.2263) (55.4723, 1.2263) (55.5882, 1.2076) (55.6409, 1.1736) knots 0 0 0 1 2 2 2
  spline S189 degree 2 poles (55.6409, 1.1736) (55.6936, 1.1396) (55.7543, 1.0334) (55.7543, 0.9548) knots 0 0 0 1 2 2 2
  spline S190 degree 2 poles (55.7543, 0.9548) (55.7543, 0.8454) (55.6425, 0.6971) (55.5469, 0.6614) knots 0 0 0 1 2 2 2
  line L290 (55.5469, 0.6614) -> (55.9026, 0.2263)
  spline S191 degree 2 poles (55.6158, 0.9443) (55.6158, 0.988) (55.585, 1.0553) (55.5525, 1.0772) knots 0 0 0 1 2 2 2
  spline S192 degree 2 poles (55.5525, 1.0772) (55.5242, 1.0958) (55.4488, 1.1112) (55.3937, 1.1112) knots 0 0 0 1 2 2 2
  line L291 (55.3937, 1.1112) -> (55.2616, 1.1112)
  line L292 (55.2616, 1.1112) -> (55.2616, 0.7352)
  line L293 (55.2616, 0.7352) -> (55.3783, 0.7352)
  spline S193 degree 2 poles (55.3783, 0.7352) (55.4359, 0.7352) (55.5274, 0.7554) (55.559, 0.787) knots 0 0 0 1 2 2 2
  spline S194 degree 2 poles (55.559, 0.787) (55.5882, 0.8146) (55.6158, 0.8924) (55.6158, 0.9443) knots 0 0 0 1 2 2 2
  line L294 (56.5801, 1.1079) -> (56.1149, 1.1079)
  line L295 (56.1149, 1.1079) -> (56.1149, 0.8259)
  line L296 (56.1149, 0.8259) -> (56.5606, 0.8259)
  line L297 (56.5606, 0.8259) -> (56.5606, 0.7076)
  line L298 (56.5606, 0.7076) -> (56.1149, 0.7076)
  line L299 (56.1149, 0.7076) -> (56.1149, 0.2263)
  line L300 (56.1149, 0.2263) -> (55.982, 0.2263)
  line L301 (55.982, 0.2263) -> (55.982, 1.2263)
  line L302 (55.982, 1.2263) -> (56.5801, 1.2263)
  line L303 (56.5801, 1.2263) -> (56.5801, 1.1079)
  line L304 (57.2973, 1.1079) -> (56.8321, 1.1079)
  line L305 (56.8321, 1.1079) -> (56.8321, 0.8259)
  line L306 (56.8321, 0.8259) -> (57.2778, 0.8259)
  line L307 (57.2778, 0.8259) -> (57.2778, 0.7076)
  line L308 (57.2778, 0.7076) -> (56.8321, 0.7076)
  line L309 (56.8321, 0.7076) -> (56.8321, 0.2263)
  line L310 (56.8321, 0.2263) -> (56.6992, 0.2263)
  line L311 (56.6992, 0.2263) -> (56.6992, 1.2263)
  line L312 (56.6992, 1.2263) -> (57.2973, 1.2263)
  line L313 (57.2973, 1.2263) -> (57.2973, 1.1079)
  spline S195 degree 2 poles (51.4737, 0.2085) (51.3675, 0.2085) (51.1917, 0.2734) (51.1285, 0.339) knots 0 0 0 1 2 2 2
  spline S196 degree 2 poles (51.1285, 0.339) (51.0653, 0.4055) (50.998, 0.6016) (50.998, 0.7288) knots 0 0 0 1 2 2 2
  spline S197 degree 2 poles (50.998, 0.7288) (50.998, 0.8495) (51.0661, 1.0408) (51.1293, 1.1089) knots 0 0 0 1 2 2 2
  spline S198 degree 2 poles (51.1293, 1.1089) (51.1901, 1.1745) (51.3684, 1.2458) (51.4745, 1.2458) knots 0 0 0 1 2 2 2
  spline S199 degree 2 poles (51.4745, 1.2458) (51.5256, 1.2458) (51.618, 1.2312) (51.6601, 1.2183) knots 0 0 0 1 2 2 2
  spline S200 degree 2 poles (51.6601, 1.2183) (51.6941, 1.2085) (51.7768, 1.1729) (51.8019, 1.1599) knots 0 0 0 1 2 2 2
  line L314 (51.8019, 1.1599) -> (51.8019, 0.9995)
  line L315 (51.8019, 0.9995) -> (51.7906, 0.9995)
  spline S201 degree 2 poles (51.7906, 0.9995) (51.7654, 1.0213) (51.7128, 1.061) (51.6641, 1.0837) knots 0 0 0 1 2 2 2
  spline S202 degree 2 poles (51.6641, 1.0837) (51.6236, 1.104) (51.5191, 1.1307) (51.4591, 1.1307) knots 0 0 0 1 2 2 2
  spline S203 degree 2 poles (51.4591, 1.1307) (51.3149, 1.1307) (51.1366, 0.9136) (51.1366, 0.7328) knots 0 0 0 1 2 2 2
  spline S204 degree 2 poles (51.1366, 0.7328) (51.1366, 0.6324) (51.1836, 0.4816) (51.2282, 0.4298) knots 0 0 0 1 2 2 2
  spline S205 degree 2 poles (51.2282, 0.4298) (51.2711, 0.3779) (51.3927, 0.3236) (51.4688, 0.3236) knots 0 0 0 1 2 2 2
  spline S206 degree 2 poles (51.4688, 0.3236) (51.5248, 0.3236) (51.6366, 0.3398) (51.6747, 0.356) knots 0 0 0 1 2 2 2
  line L316 (51.6747, 0.356) -> (51.6747, 0.6145)
  line L317 (51.6747, 0.6145) -> (51.4429, 0.6145)
  line L318 (51.4429, 0.6145) -> (51.4429, 0.7312)
  line L319 (51.4429, 0.7312) -> (51.806, 0.7312)
  line L320 (51.806, 0.7312) -> (51.806, 0.2944)
  spline S207 degree 2 poles (51.806, 0.2944) (51.7808, 0.2831) (51.6949, 0.2482) (51.6585, 0.2377) knots 0 0 0 1 2 2 2
  spline S208 degree 2 poles (51.6585, 0.2377) (51.609, 0.2231) (51.5296, 0.2085) (51.4737, 0.2085) knots 0 0 0 1 2 2 2
  line L321 (52.6885, 0.228) -> (52.5393, 0.228)
  line L322 (52.5393, 0.228) -> (52.0969, 1.0902)
  line L323 (52.0969, 1.0902) -> (52.0969, 0.228)
  line L324 (52.0969, 0.228) -> (51.9729, 0.228)
  line L325 (51.9729, 0.228) -> (51.9729, 1.228)
  line L326 (51.9729, 1.228) -> (52.1617, 1.228)
  line L327 (52.1617, 1.228) -> (52.5645, 0.4363)
  line L328 (52.5645, 0.4363) -> (52.5645, 1.228)
  line L329 (52.5645, 1.228) -> (52.6885, 1.228)
  line L330 (52.6885, 1.228) -> (52.6885, 0.228)
  spline S209 degree 2 poles (53.6795, 0.7272) (53.6795, 0.5902) (53.5685, 0.3698) (53.4753, 0.3082) knots 0 0 0 1 2 2 2
  spline S210 degree 2 poles (53.4753, 0.3082) (53.3992, 0.2604) (53.2428, 0.228) (53.1212, 0.228) knots 0 0 0 1 2 2 2
  line L331 (53.1212, 0.228) -> (52.891, 0.228)
  line L332 (52.891, 0.228) -> (52.891, 1.228)
  line L333 (52.891, 1.228) -> (53.1188, 1.228)
  spline S211 degree 2 poles (53.1188, 1.228) (53.2598, 1.228) (53.4202, 1.1858) (53.4769, 1.1486) knots 0 0 0 1 2 2 2
  spline S212 degree 2 poles (53.4769, 1.1486) (53.5734, 1.0846) (53.6795, 0.873) (53.6795, 0.7272) knots 0 0 0 1 2 2 2
  spline S213 degree 2 poles (53.541, 0.7288) (53.541, 0.8439) (53.4648, 1.0068) (53.3894, 1.0529) knots 0 0 0 1 2 2 2
  spline S214 degree 2 poles (53.3894, 1.0529) (53.3359, 1.0846) (53.2152, 1.1129) (53.1252, 1.1129) knots 0 0 0 1 2 2 2
  line L334 (53.1252, 1.1129) -> (53.0239, 1.1129)
  line L335 (53.0239, 1.1129) -> (53.0239, 0.3431)
  line L336 (53.0239, 0.3431) -> (53.1252, 0.3431)
  spline S215 degree 2 poles (53.1252, 0.3431) (53.2136, 0.3431) (53.3473, 0.3714) (53.4016, 0.4095) knots 0 0 0 1 2 2 2
  spline S216 degree 2 poles (53.4016, 0.4095) (53.4713, 0.4565) (53.541, 0.6121) (53.541, 0.7288) knots 0 0 0 1 2 2 2
  line L337 (48.7187, 0.1993) -> (48.2308, 0.1993)
  line L338 (48.2308, 0.1993) -> (48.2308, 0.3014)
  line L339 (48.2308, 0.3014) -> (48.4123, 0.3014)
  line L340 (48.4123, 0.3014) -> (48.4123, 0.9716)
  line L341 (48.4123, 0.9716) -> (48.2308, 0.9716)
  line L342 (48.2308, 0.9716) -> (48.2308, 1.0632)
  spline S217 degree 2 poles (48.2308, 1.0632) (48.3337, 1.0632) (48.431, 1.1215) (48.4375, 1.2026) knots 0 0 0 1 2 2 2
  line L343 (48.4375, 1.2026) -> (48.5412, 1.2026)
  line L344 (48.5412, 1.2026) -> (48.5412, 0.3014)
  line L345 (48.5412, 0.3014) -> (48.7187, 0.3014)
  line L346 (48.7187, 0.3014) -> (48.7187, 0.1993)
  spline S218 degree 2 poles (49.1725, 1.1045) (49.136, 1.1045) (49.0639, 1.0867) (49.029, 1.0729) knots 0 0 0 1 2 2 2
  spline S219 degree 2 poles (49.029, 1.0729) (48.9966, 1.0591) (48.9488, 1.03) (48.9302, 1.017) knots 0 0 0 1 2 2 2
  line L347 (48.9302, 1.017) -> (48.9221, 1.017)
  line L348 (48.9221, 1.017) -> (48.9221, 1.1588)
  spline S220 degree 2 poles (48.9221, 1.1588) (48.9658, 1.1823) (49.1157, 1.2204) (49.183, 1.2204) knots 0 0 0 1 2 2 2
  spline S221 degree 2 poles (49.183, 1.2204) (49.2511, 1.2204) (49.3524, 1.1928) (49.3937, 1.1637) knots 0 0 0 1 2 2 2
  spline S222 degree 2 poles (49.3937, 1.1637) (49.4375, 1.1321) (49.4828, 1.0405) (49.4828, 0.9789) knots 0 0 0 1 2 2 2
  spline S223 degree 2 poles (49.4828, 0.9789) (49.4828, 0.8962) (49.3742, 0.7714) (49.2981, 0.7552) knots 0 0 0 1 2 2 2
  line L349 (49.2981, 0.7552) -> (49.2981, 0.7455)
  spline S224 degree 2 poles (49.2981, 0.7455) (49.3297, 0.739) (49.4018, 0.7099) (49.4326, 0.6807) knots 0 0 0 1 2 2 2
  spline S225 degree 2 poles (49.4326, 0.6807) (49.4634, 0.6523) (49.5023, 0.5616) (49.5023, 0.4959) knots 0 0 0 1 2 2 2
  spline S226 degree 2 poles (49.5023, 0.4959) (49.5023, 0.4287) (49.4561, 0.3144) (49.414, 0.2706) knots 0 0 0 1 2 2 2
  spline S227 degree 2 poles (49.414, 0.2706) (49.3702, 0.2253) (49.2462, 0.1782) (49.1676, 0.1782) knots 0 0 0 1 2 2 2
  spline S228 degree 2 poles (49.1676, 0.1782) (49.0922, 0.1782) (48.9447, 0.2147) (48.8945, 0.2398) knots 0 0 0 1 2 2 2
  line L350 (48.8945, 0.2398) -> (48.8945, 0.3817)
  line L351 (48.8945, 0.3817) -> (48.9042, 0.3817)